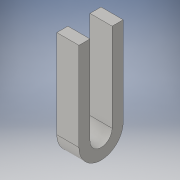
# Autodesk Inventor part: U_bolt
Saved by Autodesk Inventor 2016 SP1 (Build 200210100, 210)
## iProperties
Created: 2016-02-05
Part Number: U_bolt
Material: Generic
Document SubType Name: Modeling
Designer: steele
Density: 1 g/cm^3
Appearance: Default
Author: steele
Autodesk Inventor part; units mm, degrees
ref_plane "YZ Plane" through (0, 0, 0) normal (1, 0, 0) x (0, 1, 0)
ref_plane "XZ Plane" through (0, 0, 0) normal (0, 1, 0) x (-1, 0, 0)
ref_plane "XY Plane" through (0, 0, 0) normal (0, 0, 1) x (1, 0, 0)
sketch "Sketch1" plane through (0, 0, 0) normal (1, 0, 0) x (0, 1, 0)
  arc A0 (0, 6.35) -> (0, -6.35) centre (0, 0) ccw
  arc A1 (0, 12.7) -> (0, -12.7) centre (0, 0) ccw
  line L0 (0, 12.7) -> (50.8, 12.7)
  line L1 (0, -12.7) -> (50.8, -12.7)
  line L2 (0, 6.35) -> (50.8, 6.35)
  line L3 (0, -6.35) -> (50.8, -6.35)
  line L4 (50.8, -6.35) -> (50.8, -12.7)
  line L5 (50.8, 12.7) -> (50.8, 6.35)
  dimension "d0" = 12.7
  dimension "d1" = 25.4
  dimension "d2" = 50.8
  constraints: 12 end point, 4 horizontal, 4 point on circle, 2 centre point, 2 coincident, 1 collinear, 1 perpendicular
  measures "d0" diameter of A0
  measures "d1" diameter of A1
  measures "d2" distance of L0.start L0.end
extrude "Extrusion1" add sketch "Sketch1" along normal mid plane 12.7
body "Solid1"
